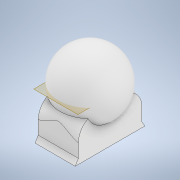
# Autodesk Inventor part: round_finger_tip_flex_smaller_holes
Saved by Autodesk Inventor 2021.3 (Build 253353000, 353)
## iProperties
Created: 2022-05-03
Part Number: round_finger_tip_flex_smaller_holes
Material: ABS Plastic
Document SubType Name: Modeling
Designer: Lucky7Chess
Density: 1.06 g/cm^3
Appearance: Smooth - White
Mass: 13.5532 g
Surface Area: 48.1491 cm^2
Volume: 12.786 cm^3
Author: Lucky7Chess
Autodesk Inventor part; units mm, degrees
ref_plane "YZ Plane" through (0, 0, 0) normal (1, 0, 0) x (0, 1, 0)
ref_plane "XY Plane" through (0, 0, 0) normal (0, 0, 1) x (1, 0, 0)
sketch "Sketch1" plane through (0, 0, 0) normal (0, 1, 0) x (-1, 0, 0)
  line L0 (0, 0) -> (-19, 0)
  line L1 (-19, 0) -> (-19, -33)
  line L2 (-19, -33) -> (0, -33)
  line L3 (0, -33) -> (0, 0)
  point P0 (0, 0)
  dimension "d0" = 19
  dimension "d1" = 33
  dimension "d27" = 0
  dimension "d28" = 0
  constraints: 8 end point, 2 parallel, 1 horizontal, 1 perpendicular
  measures "d0" distance of L2.end L1.end
  measures "d1" distance of L2.end L0.start
  measures "d27" distance of L0.start point (0, 0)
  measures "d28" distance from line of point (0, 0) L3
ref_plane "Work Plane1" through (0, 2.5, 0) normal (0, 1, 0) x (-1, 0, 0)
sketch "Sketch3" plane through (0, 2.5, 0) normal (0, 1, 0) x (-1, 0, 0)
  line L0 (0, -1.5) -> (-19, -1.5)
  line L1 (-19, -1.5) -> (-19, -31.5)
  line L2 (-19, -31.5) -> (0, -31.5)
  line L3 (0, -31.5) -> (0, -1.5)
  point P0 (0, 0)
  dimension "d29" = 19
  dimension "d30" = 30
  dimension "d31" = 1.5
  constraints: 8 end point, 2 parallel, 1 horizontal, 1 perpendicular
  measures "d29" distance of L2.end L1.end
  measures "d30" distance between parallel lines of L2 L0
  measures "d31" distance from line of point (0, 0) L0
sketch "Sketch4" plane through (0, 0, 0) normal (0, 1, 0) x (-1, 0, 0)
  line L0 (0, 0) -> (-19, 0)
  line L1 (-19, 0) -> (-19, -33)
  line L2 (-19, -33) -> (0, -33)
  line L3 (0, -33) -> (0, 0)
  circle A0 centre (-3.5, -16.5) radius 1.5
  circle A1 centre (-15.5, -16.5) radius 1.5
  circle A2 centre (-12.5, -7.5) radius 1.5
  circle A3 centre (-6.5, -7.5) radius 1.5
  circle A4 centre (-6.5, -25.5) radius 1.5
  circle A5 centre (-12.5, -25.5) radius 1.5
  point P0 (0, 0)
  dimension "d32" = 19
  dimension "d33" = 33
  dimension "d34" = 3
  dimension "d35" = 3
  dimension "d36" = 3
  dimension "d37" = 3
  dimension "d38" = 3
  dimension "d39" = 3
  dimension "d40" = 3.5
  dimension "d41" = 3.5
  dimension "d42" = 16.5
  dimension "d43" = 16.5
  dimension "d44" = 7.5
  dimension "d45" = 7.5
  dimension "d46" = 7.5
  dimension "d47" = 7.5
  dimension "d48" = 6.5
  dimension "d49" = 6.5
  dimension "d50" = 6.5
  dimension "d51" = 6.5
  dimension "d52" = 0
  dimension "d53" = 0
  constraints: 8 end point, 6 centre point, 2 parallel, 1 horizontal, 1 perpendicular
  measures "d32" distance of L2.end L1.end
  measures "d33" distance of L2.end L0.start
  measures "d34" diameter of A0
  measures "d35" diameter of A1
  measures "d36" diameter of A2
  measures "d37" diameter of A3
  measures "d38" diameter of A4
  measures "d39" diameter of A5
  measures "d40" distance from line of L3 A0.centre
  measures "d41" distance from line of L1 A1.centre
  measures "d42" distance from line of L2 A0.centre
  measures "d43" distance from line of L2 A1.centre
  measures "d44" distance from line of L0 A2.centre
  measures "d45" distance from line of L0 A3.centre
  measures "d46" distance from line of L2 A4.centre
  measures "d47" distance from line of L2 A5.centre
  measures "d48" distance from line of L3 A3.centre
  measures "d49" distance from line of L1 A2.centre
  measures "d50" distance from line of L3 A4.centre
  measures "d51" distance from line of L1 A5.centre
  measures "d52" distance of L0.start point (0, 0)
  measures "d53" distance from line of point (0, 0) L3
loft "base" add profiles "Sketch1", "Sketch3"
sketch "Sketch14" plane through (0, 2.5, -1.5) normal (0, 1, 0) x (1, 0, 0)
  line L0 (19, 30) -> (0, 30) projected
  line L1 (0, -1.5) -> (0, 0) projected
  line L2 (19, 30) -> (0, 30)
  line L3 (0, 30) -> (0, 0)
  line L4 (0, 0) -> (19, 0)
  line L5 (19, 0) -> (19, 30)
  constraints: 8 end point, 2 parallel, 1 horizontal, 1 perpendicular
extrude "Extrusion8" add sketch "Sketch14" along normal blind 14
extrude "brass_insert_holes" cut sketch "Sketch4" along normal blind 20 contours A0 | A1 | A2 | A3 | A4 | A5
ref_plane "Work Plane2" through (0, 21.5, -1.5) normal (0, 1, 0) x (1, 0, 0)
sketch "Sketch15" plane through (0, 21.5, -1.5) normal (0, 1, 0) x (1, 0, 0)
  line L0 (19, 30) -> (0, 30) projected
  line L1 (0, 0) -> (19, 0) projected
  arc A0 (9.5, 30) -> (9.5, 0) centre (9.5, 15) ccw
  line L2 (9.5, 30) -> (9.5, 0)
  point P0 (0, -1.5)
  constraints: 2 end point, 2 midpoint, 2 point on circle, 1 centre point, 1 perpendicular
revolve "Revolution1" add sketch "Sketch15" angle 360 about axis through (9.5, 21.5, -31.5) along (0, 0, -1)
fillet "Fillet4" radius 8 2 edges at (9.5, 16.5, -1.5) (9.5, 16.5, -31.5)
body "Solid1"
